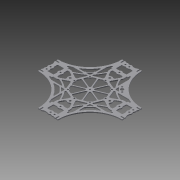
# Autodesk Inventor part: Middle Plate Over
Saved by Autodesk Inventor 2014 SP1 (Build 180222100, 222)
## iProperties
Created: 2014-07-28
Part Number: Middle Plate Over
Material: Generic
Document SubType Name: Modeling
Designer: Ryan
Density: 1 g/cm^3
Appearance: Default
Mass: 14.8472 g
Surface Area: 207.77 cm^2
Volume: 14.8472 cm^3
Author: Ryan
Autodesk Inventor part; units mm, degrees
(part 1 of 2)
ref_plane "YZ Plane" through (0, 0, 0) normal (1, 0, 0) x (0, 1, 0)
ref_plane "XZ Plane" through (0, 0, 0) normal (0, 1, 0) x (-1, 0, 0)
ref_plane "XY Plane" through (0, 0, 0) normal (0, 0, 1) x (1, 0, 0)
sketch "Middle Plate Over" plane through (0, 0, 0) normal (0, 0, 1) x (1, 0, 0)
  circle A0 centre (54.1802, 86) radius 1.6
  circle A1 centre (63.5, 108.5) radius 1.6
  circle A2 centre (86, 117.8198) radius 1.6
  circle A3 centre (108.5, 108.5) radius 1.6
  circle A4 centre (117.8198, 86) radius 1.6
  circle A5 centre (108.5, 63.5) radius 1.6
  circle A6 centre (63.5, 63.5) radius 1.6
  circle A7 centre (86, 54.1802) radius 1.6
  arc A8 (56.1767, 84.1823) -> (56.1767, 87.8177) centre (54.1802, 86) ccw
  arc A9 (55.8078, 89.9295) -> (56.1767, 87.8177) centre (57.6556, 89.1641) ccw
  arc A10 (56.1767, 84.1823) -> (55.8078, 82.0705) centre (57.6556, 82.8359) ccw
  arc A11 (63.6264, 105.803) -> (66.197, 108.3735) centre (63.5, 108.5) ccw
  arc A12 (63.6264, 105.803) -> (61.8724, 104.5705) centre (63.7201, 103.8052) ccw
  arc A13 (67.4295, 110.1276) -> (66.197, 108.3735) centre (68.1948, 108.2799) ccw
  arc A14 (84.1823, 115.8233) -> (87.8177, 115.8233) centre (86, 117.8198) ccw
  arc A15 (89.9295, 116.1922) -> (87.8177, 115.8233) centre (89.1641, 114.3444) ccw
  arc A16 (84.1823, 115.8233) -> (82.0705, 116.1922) centre (82.8359, 114.3444) ccw
  arc A17 (105.803, 108.3735) -> (108.3735, 105.803) centre (108.5, 108.5) ccw
  arc A18 (110.1276, 104.5705) -> (108.3735, 105.803) centre (108.2799, 103.8052) ccw
  arc A19 (105.803, 108.3735) -> (104.5705, 110.1276) centre (103.8052, 108.2799) ccw
  arc A20 (115.8233, 87.8177) -> (115.8233, 84.1823) centre (117.8198, 86) ccw
  arc A21 (116.1922, 82.0705) -> (115.8233, 84.1823) centre (114.3444, 82.8359) ccw
  arc A22 (115.8233, 87.8177) -> (116.1922, 89.9295) centre (114.3444, 89.1641) ccw
  arc A23 (66.197, 63.6265) -> (63.6264, 66.197) centre (63.5, 63.5) ccw
  arc A24 (61.8724, 67.4295) -> (63.6264, 66.197) centre (63.7201, 68.1948) ccw
  arc A25 (66.197, 63.6265) -> (67.4295, 61.8724) centre (68.1948, 63.7201) ccw
  arc A26 (87.8177, 56.1767) -> (84.1823, 56.1767) centre (86, 54.1802) ccw
  arc A27 (82.0705, 55.8078) -> (84.1823, 56.1767) centre (82.8359, 57.6556) ccw
  arc A28 (87.8177, 56.1767) -> (89.9295, 55.8078) centre (89.1641, 57.6556) ccw
  arc A29 (108.3735, 66.197) -> (105.803, 63.6265) centre (108.5, 63.5) ccw
  arc A30 (104.5705, 61.8724) -> (105.803, 63.6265) centre (103.8052, 63.7201) ccw
  arc A31 (108.3735, 66.197) -> (110.1276, 67.4295) centre (108.2799, 68.1948) ccw
  line L0 (55.8078, 82.0705) -> (61.8724, 67.4295)
  line L1 (67.4295, 61.8724) -> (82.0705, 55.8078)
  line L2 (89.9295, 55.8078) -> (104.5705, 61.8724)
  line L3 (110.1276, 67.4295) -> (116.1922, 82.0705)
  line L4 (116.1922, 89.9295) -> (110.1276, 104.5705)
  line L5 (104.5705, 110.1276) -> (89.9295, 116.1922)
  line L6 (82.0705, 116.1922) -> (67.4295, 110.1276)
  line L7 (61.8724, 104.5705) -> (55.8078, 89.9295)
  line L8 (0, 99.484) -> (0, 101)
  arc A32 (0, 99.484) -> (0.217, 98.5779) centre (2, 99.484) ccw
  line L9 (0, 101) -> (6.5, 101)
  line L10 (6.5, 101) -> (6.5, 103.2)
  line L11 (6.5, 103.2) -> (0, 103.2)
  line L12 (0, 103.2) -> (0, 106.2)
  line L13 (71, 172) -> (71, 165.5)
  line L14 (71, 165.5) -> (68.8, 165.5)
  line L15 (68.8, 165.5) -> (68.8, 172)
  line L16 (68.8, 172) -> (65.8, 172)
  arc A33 (0, 106.2) -> (65.8, 172) centre (0, 172) ccw
  line L17 (101, 172) -> (101, 165.5)
  line L18 (101, 165.5) -> (103.2, 165.5)
  line L19 (103.2, 165.5) -> (103.2, 172)
  line L20 (103.2, 172) -> (106.2, 172)
  line L21 (172, 101) -> (165.5, 101)
  line L22 (165.5, 101) -> (165.5, 103.2)
  line L23 (165.5, 103.2) -> (172, 103.2)
  line L24 (172, 103.2) -> (172, 106.2)
  arc A34 (106.2, 172) -> (172, 106.2) centre (172, 172) ccw
  line L25 (0, 71) -> (6.5, 71)
  line L26 (6.5, 71) -> (6.5, 68.8)
  line L27 (6.5, 68.8) -> (0, 68.8)
  line L28 (0, 68.8) -> (0, 65.8)
  line L29 (71, 0) -> (71, 6.5)
  line L30 (71, 6.5) -> (68.8, 6.5)
  line L31 (68.8, 6.5) -> (68.8, 0)
  line L32 (68.8, 0) -> (65.8, 0)
  arc A35 (65.8, 0) -> (0, 65.8) centre (0, 0) ccw
  line L33 (101, 0) -> (101, 6.5)
  line L34 (101, 6.5) -> (103.2, 6.5)
  line L35 (103.2, 6.5) -> (103.2, 0)
  line L36 (103.2, 0) -> (106.2, 0)
  line L37 (172, 71) -> (165.5, 71)
  line L38 (165.5, 71) -> (165.5, 68.8)
  line L39 (165.5, 68.8) -> (172, 68.8)
  line L40 (172, 68.8) -> (172, 65.8)
  arc A36 (172, 65.8) -> (106.2, 0) centre (172, 0) ccw
  circle A37 centre (45.5084, 86) radius 2.1
  circle A38 centre (5.472, 86) radius 1.6
  circle A39 centre (25.7484, 86) radius 1.6
  line L41 (10.792, 96.8671) -> (20.4284, 96.8671)
  arc A40 (10.792, 96.8671) -> (8.892, 94.9671) centre (10.792, 94.9671) ccw
  line L42 (8.892, 94.9671) -> (8.892, 89.42)
  line L43 (22.3284, 89.42) -> (22.3284, 94.9671)
  arc A41 (22.3284, 94.9671) -> (20.4284, 96.8671) centre (20.4284, 94.9671) ccw
  line L44 (10.2433, 75.1329) -> (20.4284, 75.1329)
  line L45 (22.3284, 82.58) -> (22.3284, 77.0329)
  arc A42 (20.4284, 75.1329) -> (22.3284, 77.0329) centre (20.4284, 77.0329) ccw
  arc A43 (9.3838, 83.1636) -> (8.892, 89.42) centre (5.426, 86) ccw
  arc A44 (22.3284, 89.42) -> (22.3284, 82.58) centre (25.7484, 86) ccw
  line L46 (32.9349, 96.8671) -> (31.0684, 96.8671)
  line L47 (29.1684, 89.42) -> (29.1684, 94.9671)
  arc A45 (31.0684, 96.8671) -> (29.1684, 94.9671) centre (31.0684, 94.9671) ccw
  arc A46 (29.1684, 82.58) -> (29.1684, 89.42) centre (25.7484, 86) ccw
  line L48 (33.8405, 96.6374) -> (41.094, 92.7047)
  arc A47 (33.8405, 96.6374) -> (32.9349, 96.8671) centre (32.9349, 94.9671) ccw
  line L49 (42.0884, 91.0344) -> (42.0884, 89.42)
  arc A48 (42.0884, 91.0344) -> (41.094, 92.7047) centre (40.1884, 91.0344) ccw
  arc A49 (42.0884, 89.42) -> (42.0884, 82.58) centre (45.5084, 86) ccw
  line L50 (32.9349, 75.1329) -> (31.0684, 75.1329)
  line L51 (29.1684, 82.58) -> (29.1684, 77.0329)
  arc A50 (29.1684, 77.0329) -> (31.0684, 75.1329) centre (31.0684, 77.0329) ccw
  line L52 (33.8405, 75.3626) -> (41.094, 79.2953)
  arc A51 (32.9349, 75.1329) -> (33.8405, 75.3626) centre (32.9349, 77.0329) ccw
  line L53 (42.0884, 80.9656) -> (42.0884, 82.58)
  arc A52 (41.094, 79.2953) -> (42.0884, 80.9656) centre (40.1884, 80.9656) ccw
  circle A53 centre (126.4916, 86) radius 2.1
  circle A54 centre (146.2516, 86) radius 1.6
  line L54 (161.7567, 96.8671) -> (151.5716, 96.8671)
  line L55 (149.6716, 89.42) -> (149.6716, 94.9671)
  arc A55 (151.5716, 96.8671) -> (149.6716, 94.9671) centre (151.5716, 94.9671) ccw
  line L56 (161.208, 75.1329) -> (151.5716, 75.1329)
  line L57 (149.6716, 82.58) -> (149.6716, 77.0329)
  arc A56 (149.6716, 77.0329) -> (151.5716, 75.1329) centre (151.5716, 77.0329) ccw
  arc A57 (149.6716, 82.58) -> (149.6716, 89.42) centre (146.2516, 86) ccw
  line L58 (139.0651, 96.8671) -> (140.9316, 96.8671)
  line L59 (142.8316, 89.42) -> (142.8316, 94.9671)
  arc A58 (142.8316, 94.9671) -> (140.9316, 96.8671) centre (140.9316, 94.9671) ccw
  arc A59 (142.8316, 89.42) -> (142.8316, 82.58) centre (146.2516, 86) ccw
  line L60 (138.1595, 96.6374) -> (130.906, 92.7047)
  arc A60 (139.0651, 96.8671) -> (138.1595, 96.6374) centre (139.0651, 94.9671) ccw
  line L61 (129.9116, 91.0344) -> (129.9116, 89.42)
  arc A61 (130.906, 92.7047) -> (129.9116, 91.0344) centre (131.8116, 91.0344) ccw
  arc A62 (129.9116, 82.58) -> (129.9116, 89.42) centre (126.4916, 86) ccw
  line L62 (139.0651, 75.1329) -> (140.9316, 75.1329)
  line L63 (142.8316, 82.58) -> (142.8316, 77.0329)
  arc A63 (140.9316, 75.1329) -> (142.8316, 77.0329) centre (140.9316, 77.0329) ccw
  line L64 (138.1595, 75.3626) -> (130.906, 79.2953)
  arc A64 (138.1595, 75.3626) -> (139.0651, 75.1329) centre (139.0651, 77.0329) ccw
  line L65 (129.9116, 80.9656) -> (129.9116, 82.58)
  arc A65 (129.9116, 80.9656) -> (130.906, 79.2953) centre (131.8116, 80.9656) ccw
  circle A66 centre (86, 126.4916) radius 2.1
  circle A67 centre (86, 146.2516) radius 1.6
  line L66 (75.1329, 161.7567) -> (75.1329, 151.5716)
  line L67 (82.58, 149.6716) -> (77.0329, 149.6716)
  arc A68 (75.1329, 151.5716) -> (77.0329, 149.6716) centre (77.0329, 151.5716) ccw
  line L68 (96.8671, 161.208) -> (96.8671, 151.5716)
  line L69 (89.42, 149.6716) -> (94.9671, 149.6716)
  arc A69 (94.9671, 149.6716) -> (96.8671, 151.5716) centre (94.9671, 151.5716) ccw
  arc A70 (89.42, 149.6716) -> (82.58, 149.6716) centre (86, 146.2516) ccw
  line L70 (75.1329, 139.0651) -> (75.1329, 140.9316)
  line L71 (82.58, 142.8316) -> (77.0329, 142.8316)
  arc A71 (77.0329, 142.8316) -> (75.1329, 140.9316) centre (77.0329, 140.9316) ccw
  arc A72 (82.58, 142.8316) -> (89.42, 142.8316) centre (86, 146.2516) ccw
  line L72 (75.3626, 138.1595) -> (79.2953, 130.906)
  arc A73 (75.1329, 139.0651) -> (75.3626, 138.1595) centre (77.0329, 139.0651) ccw
  arc A74 (96.8671, 20.4284) -> (94.9671, 22.3284) centre (94.9671, 20.4284) ccw
  line L73 (80.9656, 129.9116) -> (82.58, 129.9116)
  arc A75 (79.2953, 130.906) -> (80.9656, 129.9116) centre (80.9656, 131.8116) ccw
  arc A76 (89.42, 129.9116) -> (82.58, 129.9116) centre (86, 126.4916) ccw
  line L74 (96.8671, 139.0651) -> (96.8671, 140.9316)
  line L75 (89.42, 142.8316) -> (94.9671, 142.8316)
  arc A77 (96.8671, 140.9316) -> (94.9671, 142.8316) centre (94.9671, 140.9316) ccw
  line L76 (96.6374, 138.1595) -> (92.7047, 130.906)
  line L77 (96.8671, 32.9349) -> (96.8671, 31.0684)
  arc A78 (96.6374, 138.1595) -> (96.8671, 139.0651) centre (94.9671, 139.0651) ccw
  line L78 (91.0344, 129.9116) -> (89.42, 129.9116)
  arc A79 (91.0344, 129.9116) -> (92.7047, 130.906) centre (91.0344, 131.8116) ccw
  circle A80 centre (86, 45.5084) radius 2.1
  circle A81 centre (86, 25.7484) radius 1.6
  line L79 (96.8671, 10.2433) -> (96.8671, 20.4284)
  line L80 (89.42, 22.3284) -> (94.9671, 22.3284)
  line L81 (75.1329, 10.792) -> (75.1329, 20.4284)
  arc A82 (92.7047, 41.094) -> (91.0344, 42.0884) centre (91.0344, 40.1884) ccw
  line L82 (82.58, 22.3284) -> (77.0329, 22.3284)
  line L83 (82.58, 29.1684) -> (77.0329, 29.1684)
  arc A83 (77.0329, 22.3284) -> (75.1329, 20.4284) centre (77.0329, 20.4284) ccw
  arc A84 (82.58, 22.3284) -> (89.42, 22.3284) centre (86, 25.7484) ccw
  line L84 (80.9656, 42.0884) -> (82.58, 42.0884)
  line L85 (89.42, 29.1684) -> (94.9671, 29.1684)
  arc A85 (94.9671, 29.1684) -> (96.8671, 31.0684) centre (94.9671, 31.0684) ccw
  arc A86 (89.42, 29.1684) -> (82.58, 29.1684) centre (86, 25.7484) ccw
  line L86 (96.6374, 33.8405) -> (92.7047, 41.094)
  arc A87 (96.8671, 32.9349) -> (96.6374, 33.8405) centre (94.9671, 32.9349) ccw
  line L87 (91.0344, 42.0884) -> (89.42, 42.0884)
  arc A88 (82.58, 42.0884) -> (89.42, 42.0884) centre (86, 45.5084) ccw
  line L88 (75.1329, 32.9349) -> (75.1329, 31.0684)
  arc A89 (75.1329, 31.0684) -> (77.0329, 29.1684) centre (77.0329, 31.0684) ccw
  arc A90 (80.9656, 42.0884) -> (79.2953, 41.094) centre (80.9656, 40.1884) ccw
  line L89 (75.3626, 33.8405) -> (79.2953, 41.094)
  arc A91 (75.3626, 33.8405) -> (75.1329, 32.9349) centre (77.0329, 32.9349) ccw
  line L90 (2.052, 94.4881) -> (2.052, 89.42)
  arc A92 (2.052, 89.42) -> (1.5587, 83.1656) centre (5.518, 86) ccw
  line L91 (0.217, 98.5779) -> (1.835, 95.3941)
  arc A93 (2.052, 94.4881) -> (1.835, 95.3941) centre (0.052, 94.4881) ccw
  arc A94 (0.217, 73.4221) -> (0, 72.516) centre (2, 72.516) ccw
  line L92 (0.217, 73.4221) -> (0.8629, 74.6931)
  line L93 (0, 71) -> (0, 72.516)
  circle A95 centre (5.47, 78) radius 1.6
  arc A96 (9.7945, 75.8533) -> (9.3832, 80.8344) centre (5.424, 78) ccw
  arc A97 (9.7945, 75.8533) -> (10.2433, 75.1329) centre (10.2433, 75.6329) ccw
  arc A98 (9.3838, 83.1636) -> (9.3832, 80.8344) centre (11.0095, 81.9986) ccw
  arc A99 (1.5581, 80.8364) -> (0.9538, 76.2982) centre (5.516, 78) ccw
  arc A100 (1.5581, 80.8364) -> (1.5587, 83.1656) centre (-0.0675, 82.0014) ccw
  arc A101 (0.8629, 74.6931) -> (0.9538, 76.2982) centre (-0.9201, 75.5992) ccw
  line L94 (172, 72.516) -> (172, 71)
  arc A102 (172, 72.516) -> (171.783, 73.4221) centre (170, 72.516) ccw
  circle A103 centre (166.528, 86) radius 1.6
  arc A104 (161.208, 75.1329) -> (163.108, 77.0329) centre (161.208, 77.0329) ccw
  line L95 (163.108, 77.0329) -> (163.108, 82.58)
  arc A105 (162.6162, 88.8364) -> (163.108, 82.58) centre (166.574, 86) ccw
  line L96 (169.948, 77.5119) -> (169.948, 82.58)
  arc A106 (169.948, 82.58) -> (170.4413, 88.8344) centre (166.482, 86) ccw
  line L97 (171.783, 73.4221) -> (170.165, 76.6059)
  arc A107 (169.948, 77.5119) -> (170.165, 76.6059) centre (171.948, 77.5119) ccw
  arc A108 (171.783, 98.5779) -> (172, 99.484) centre (170, 99.484) ccw
  line L98 (171.783, 98.5779) -> (171.1371, 97.3069)
  line L99 (172, 101) -> (172, 99.484)
  circle A109 centre (166.53, 94) radius 1.6
  arc A110 (162.2055, 96.1467) -> (162.6167, 91.1656) centre (166.576, 94) ccw
  arc A111 (162.2055, 96.1467) -> (161.7567, 96.8671) centre (161.7567, 96.3671) ccw
  arc A112 (162.6162, 88.8364) -> (162.6167, 91.1656) centre (160.9905, 90.0014) ccw
  arc A113 (170.4419, 91.1636) -> (171.0462, 95.7018) centre (166.484, 94) ccw
  arc A114 (170.4419, 91.1636) -> (170.4413, 88.8344) centre (172.0675, 89.9986) ccw
  arc A115 (171.1371, 97.3069) -> (171.0462, 95.7018) centre (172.92, 96.4008) ccw
  line L100 (72.516, 0) -> (71, 0)
  arc A116 (72.516, 0) -> (73.4221, 0.217) centre (72.516, 2) ccw
  circle A117 centre (86, 5.472) radius 1.6
  arc A118 (75.1329, 10.792) -> (77.0329, 8.892) centre (77.0329, 10.792) ccw
  line L101 (77.0329, 8.892) -> (82.58, 8.892)
  arc A119 (88.8364, 9.3838) -> (82.58, 8.892) centre (86, 5.426) ccw
  line L102 (77.5119, 2.052) -> (82.58, 2.052)
  arc A120 (82.58, 2.052) -> (88.8344, 1.5587) centre (86, 5.518) ccw
  line L103 (73.4221, 0.217) -> (76.6059, 1.835)
  arc A121 (77.5119, 2.052) -> (76.6059, 1.835) centre (77.5119, 0.052) ccw
  arc A122 (98.5779, 0.217) -> (99.484, 0) centre (99.484, 2) ccw
  line L104 (98.5779, 0.217) -> (97.3069, 0.8629)
  line L105 (101, 0) -> (99.484, 0)
  circle A123 centre (94, 5.47) radius 1.6
  arc A124 (96.1467, 9.7945) -> (91.1656, 9.3833) centre (94, 5.424) ccw
  arc A125 (96.1467, 9.7945) -> (96.8671, 10.2433) centre (96.3671, 10.2433) ccw
  arc A126 (88.8364, 9.3838) -> (91.1656, 9.3833) centre (90.0014, 11.0095) ccw
  arc A127 (91.1636, 1.5581) -> (95.7018, 0.9538) centre (94, 5.516) ccw
  arc A128 (91.1636, 1.5581) -> (88.8344, 1.5587) centre (89.9986, -0.0675) ccw
  arc A129 (97.3069, 0.8629) -> (95.7018, 0.9538) centre (96.4008, -0.92) ccw
  line L106 (99.484, 172) -> (101, 172)
  arc A130 (99.484, 172) -> (98.5779, 171.783) centre (99.484, 170) ccw
  circle A131 centre (86, 166.528) radius 1.6
  arc A132 (96.8671, 161.208) -> (94.9671, 163.108) centre (94.9671, 161.208) ccw
  line L107 (94.9671, 163.108) -> (89.42, 163.108)
  arc A133 (83.1636, 162.6162) -> (89.42, 163.108) centre (86, 166.574) ccw
  line L108 (94.4881, 169.948) -> (89.42, 169.948)
  arc A134 (89.42, 169.948) -> (83.1656, 170.4413) centre (86, 166.482) ccw
  line L109 (98.5779, 171.783) -> (95.3941, 170.165)
  arc A135 (94.4881, 169.948) -> (95.3941, 170.165) centre (94.4881, 171.948) ccw
  arc A136 (73.4221, 171.783) -> (72.516, 172) centre (72.516, 170) ccw
  line L110 (73.4221, 171.783) -> (74.6931, 171.1371)
  line L111 (71, 172) -> (72.516, 172)
  circle A137 centre (78, 166.53) radius 1.6
  arc A138 (75.8533, 162.2055) -> (80.8344, 162.6167) centre (78, 166.576) ccw
  arc A139 (75.8533, 162.2055) -> (75.1329, 161.7567) centre (75.6329, 161.7567) ccw
  arc A140 (83.1636, 162.6162) -> (80.8344, 162.6167) centre (81.9986, 160.9905) ccw
  arc A141 (80.8364, 170.4419) -> (76.2982, 171.0462) centre (78, 166.484) ccw
  arc A142 (80.8364, 170.4419) -> (83.1656, 170.4413) centre (82.0014, 172.0675) ccw
  arc A143 (74.6931, 171.1371) -> (76.2982, 171.0462) centre (75.5992, 172.92) ccw
  arc A144 (38.545, 113.3432) -> (58.6568, 133.455) centre (3.1615, 168.8384) ccw
  arc A145 (38.545, 113.3432) -> (39.0827, 111.5) centre (39.0827, 112.5) ccw
  arc A146 (60.5, 132.9173) -> (58.6568, 133.455) centre (59.5, 132.9173) ccw
  line L112 (58, 111.5) -> (53.3233, 111.5)
  line L113 (48.0955, 111.5) -> (39.0827, 111.5)
  line L114 (60.5, 114) -> (60.5, 118.6767)
  line L115 (60.5, 123.9045) -> (60.5, 132.9173)
  arc A147 (58, 111.5) -> (60.5, 114) centre (58, 114) ccw
  circle A148 centre (53.1485, 53.0665) radius 3.15
  circle A149 centre (48.4963, 57.6887) radius 1.6
  circle A150 centre (57.6887, 48.4963) radius 1.6
  line L116 (63.5, 122.7047) -> (63.5, 142.036)
  arc A151 (63.7361, 116.072) -> (73.3555, 131.2701) centre (13.4685, 158.5315) ccw
  arc A152 (63.7361, 116.072) -> (63.5, 115.4267) centre (64.5, 115.4267) ccw
  arc A153 (75.1447, 131.3324) -> (73.3555, 131.2701) centre (74.2656, 130.8558) ccw
  arc A154 (63.7004, 143.0168) -> (65.9031, 148.9586) centre (3.1615, 168.8384) ccw
  arc A155 (63.7004, 143.0168) -> (63.5, 142.036) centre (66, 142.036) ccw
  arc A156 (68.8, 150.6725) -> (65.9031, 148.9586) centre (68.4135, 148.0207) ccw
  line L117 (71.3627, 138.308) -> (72.3159, 136.55)
  line L118 (71, 146.5) -> (71, 139.7379)
  arc A157 (71, 139.7379) -> (71.3627, 138.308) centre (74, 139.7379) ccw
  arc A158 (49.3372, 111.9321) -> (60.0679, 122.6628) centre (8.4853, 163.5147) ccw
  arc A159 (48.0955, 111.5) -> (49.3372, 111.9321) centre (48.0955, 113.5) ccw
  arc A160 (60.0679, 122.6628) -> (60.5, 123.9045) centre (58.5, 123.9045) ccw
  arc A161 (52.9958, 112.3778) -> (59.6222, 119.0042) centre (9.8995, 162.1005) ccw
  arc A162 (52.9958, 112.3778) -> (53.3233, 111.5) centre (53.3233, 112) ccw
  arc A163 (60.5, 118.6767) -> (59.6222, 119.0042) centre (60, 118.6767) ccw
  arc A164 (113.3432, 133.455) -> (133.455, 113.3432) centre (168.8384, 168.8384) ccw
  arc A165 (132.9173, 111.5) -> (133.455, 113.3432) centre (132.9173, 112.5) ccw
  arc A166 (113.3432, 133.455) -> (111.5, 132.9173) centre (112.5, 132.9173) ccw
  line L119 (114, 111.5) -> (118.6767, 111.5)
  line L120 (123.9045, 111.5) -> (132.9173, 111.5)
  line L121 (111.5, 114) -> (111.5, 118.6767)
  line L122 (111.5, 123.9045) -> (111.5, 132.9173)
  arc A167 (111.5, 114) -> (114, 111.5) centre (114, 114) ccw
  arc A168 (111.9321, 122.6628) -> (122.6628, 111.9321) centre (163.5147, 163.5147) ccw
  arc A169 (122.6628, 111.9321) -> (123.9045, 111.5) centre (123.9045, 113.5) ccw
  arc A170 (111.5, 123.9045) -> (111.9321, 122.6628) centre (113.5, 123.9045) ccw
  arc A171 (112.3778, 119.0042) -> (119.0041, 112.3778) centre (162.1005, 162.1005) ccw
  arc A172 (118.6767, 111.5) -> (119.0041, 112.3778) centre (118.6767, 112) ccw
  arc A173 (112.3778, 119.0042) -> (111.5, 118.6767) centre (112, 118.6767) ccw
  arc A174 (133.455, 58.6568) -> (113.3432, 38.545) centre (168.8384, 3.1616) ccw
  arc A175 (133.455, 58.6568) -> (132.9173, 60.5) centre (132.9173, 59.5) ccw
  arc A176 (111.5, 39.0827) -> (113.3432, 38.545) centre (112.5, 39.0827) ccw
  line L123 (114, 60.5) -> (118.6767, 60.5)
  line L124 (123.9045, 60.5) -> (132.9173, 60.5)
  line L125 (111.5, 58) -> (111.5, 53.3233)
  line L126 (111.5, 48.0955) -> (111.5, 39.0827)
  arc A177 (114, 60.5) -> (111.5, 58) centre (114, 58) ccw
  arc A178 (122.6628, 60.0679) -> (111.9321, 49.3372) centre (163.5147, 8.4853) ccw
  arc A179 (123.9045, 60.5) -> (122.6628, 60.0679) centre (123.9045, 58.5) ccw
  arc A180 (111.9321, 49.3372) -> (111.5, 48.0955) centre (113.5, 48.0955) ccw
  arc A181 (119.0041, 59.6222) -> (112.3778, 52.9958) centre (162.1005, 9.8995) ccw
  arc A182 (119.0041, 59.6222) -> (118.6767, 60.5) centre (118.6767, 60) ccw
  arc A183 (111.5, 53.3233) -> (112.3778, 52.9958) centre (112, 53.3233) ccw
  line L127 (58, 60.5) -> (53.3233, 60.5)
  line L128 (60.5, 58) -> (60.5, 53.3233)
  arc A184 (60.5, 58) -> (58, 60.5) centre (58, 58) ccw
  arc A185 (59.6222, 52.9958) -> (52.9958, 59.6222) centre (9.8995, 9.8995) ccw
  arc A186 (53.3233, 60.5) -> (52.9958, 59.6222) centre (53.3233, 60) ccw
  arc A187 (59.6222, 52.9958) -> (60.5, 53.3233) centre (60, 53.3233) ccw
  line L129 (75.1447, 131.3324) -> (80.089, 122.2131)
  arc A188 (78.848, 118.7118) -> (80.089, 122.2131) centre (77.8913, 121.0215) ccw
  line L130 (64.8827, 112.9272) -> (78.848, 118.7118)
  arc A189 (65.314, 122.1239) -> (72.401, 134.8209) centre (11.7536, 160.3459) ccw
  arc A190 (63.5, 122.7047) -> (65.314, 122.1239) centre (64.5, 122.7047) ccw
  arc A191 (72.401, 134.8209) -> (72.3159, 136.55) centre (70.5576, 135.5967) ccw
  line L131 (63.5, 115.4267) -> (63.5, 113.8511)
  arc A192 (63.5, 113.8511) -> (64.8827, 112.9272) centre (64.5, 113.8511) ccw
  line L132 (49.2953, 108.5) -> (29.964, 108.5)
  arc A193 (40.7299, 98.6445) -> (55.928, 108.2639) centre (13.4685, 158.5315) ccw
  arc A194 (56.5733, 108.5) -> (55.928, 108.2639) centre (56.5733, 107.5) ccw
  arc A195 (40.7299, 98.6445) -> (40.6676, 96.8553) centre (41.1442, 97.7344) ccw
  arc A196 (23.0414, 106.0969) -> (28.9832, 108.2996) centre (3.1615, 168.8384) ccw
  arc A197 (29.964, 108.5) -> (28.9832, 108.2996) centre (29.964, 106) ccw
  arc A198 (23.0414, 106.0969) -> (21.3275, 103.2) centre (23.9793, 103.5865) ccw
  line L133 (33.692, 100.6373) -> (35.45, 99.6841)
  line L134 (25.5, 101) -> (32.2621, 101)
  arc A199 (33.692, 100.6373) -> (32.2621, 101) centre (32.2621, 98) ccw
  line L135 (40.6676, 96.8553) -> (49.7869, 91.911)
  arc A200 (49.7869, 91.911) -> (53.2882, 93.152) centre (50.9785, 94.1087) ccw
  line L136 (59.0728, 107.1173) -> (53.2882, 93.152)
  arc A201 (37.1791, 99.599) -> (49.8761, 106.686) centre (11.6541, 160.2464) ccw
  arc A202 (49.8761, 106.686) -> (49.2953, 108.5) centre (49.2953, 107.5) ccw
  arc A203 (35.45, 99.6841) -> (37.1791, 99.599) centre (36.4033, 101.4424) ccw
  line L137 (56.5733, 108.5) -> (58.1489, 108.5)
  arc A204 (59.0728, 107.1173) -> (58.1489, 108.5) centre (58.1489, 107.5) ccw
  line L138 (122.7047, 63.5) -> (142.036, 63.5)
  arc A205 (131.2701, 73.3555) -> (116.072, 63.7361) centre (158.5315, 13.4685) ccw
  arc A206 (115.4267, 63.5) -> (116.072, 63.7361) centre (115.4267, 64.5) ccw
  arc A207 (131.2701, 73.3555) -> (131.3324, 75.1447) centre (130.8558, 74.2656) ccw
  arc A208 (148.9586, 65.9031) -> (143.0168, 63.7004) centre (168.8384, 3.1616) ccw
  arc A209 (142.036, 63.5) -> (143.0168, 63.7004) centre (142.036, 66) ccw
  arc A210 (148.9586, 65.9031) -> (150.6725, 68.8) centre (148.0207, 68.4135) ccw
  line L139 (138.308, 71.3627) -> (136.55, 72.3159)
  line L140 (146.5, 71) -> (139.7379, 71)
  arc A211 (138.308, 71.3627) -> (139.7379, 71) centre (139.7379, 74) ccw
  line L141 (131.3324, 75.1447) -> (122.2131, 80.089)
  arc A212 (122.2131, 80.089) -> (118.7118, 78.848) centre (121.0215, 77.8913) ccw
  line L142 (112.9272, 64.8827) -> (118.7118, 78.848)
  arc A213 (134.8209, 72.401) -> (122.1239, 65.314) centre (160.3459, 11.7536) ccw
  arc A214 (122.1239, 65.314) -> (122.7047, 63.5) centre (122.7047, 64.5) ccw
  arc A215 (136.55, 72.3159) -> (134.8209, 72.401) centre (135.5967, 70.5576) ccw
  line L143 (115.4267, 63.5) -> (113.8511, 63.5)
  arc A216 (112.9272, 64.8827) -> (113.8511, 63.5) centre (113.8511, 64.5) ccw
  line L144 (108.5, 49.2953) -> (108.5, 29.964)
  arc A217 (108.2639, 55.928) -> (98.6445, 40.7299) centre (158.5315, 13.4685) ccw
  arc A218 (108.2639, 55.928) -> (108.5, 56.5733) centre (107.5, 56.5733) ccw
  arc A219 (96.8553, 40.6676) -> (98.6445, 40.7299) centre (97.7344, 41.1442) ccw
  arc A220 (108.2996, 28.9832) -> (106.0968, 23.0414) centre (168.8384, 3.1616) ccw
  arc A221 (108.2996, 28.9832) -> (108.5, 29.964) centre (106, 29.964) ccw
  arc A222 (103.2, 21.3275) -> (106.0968, 23.0414) centre (103.5865, 23.9793) ccw
  line L145 (100.6373, 33.692) -> (99.6841, 35.45)
  line L146 (101, 25.5) -> (101, 32.2621)
  arc A223 (101, 32.2621) -> (100.6373, 33.692) centre (98, 32.2621) ccw
  line L147 (96.8553, 40.6676) -> (91.911, 49.7869)
  arc A224 (93.152, 53.2882) -> (91.911, 49.7869) centre (94.1087, 50.9785) ccw
  line L148 (107.1173, 59.0728) -> (93.152, 53.2882)
  arc A225 (106.686, 49.8761) -> (99.599, 37.1791) centre (160.2464, 11.6541) ccw
  arc A226 (108.5, 49.2953) -> (106.686, 49.8761) centre (107.5, 49.2953) ccw
  arc A227 (99.599, 37.1791) -> (99.6841, 35.45) centre (101.4423, 36.4033) ccw
  line L149 (108.5, 56.5733) -> (108.5, 58.1489)
  arc A228 (108.5, 58.1489) -> (107.1173, 59.0728) centre (107.5, 58.1489) ccw
  line L150 (63.5, 49.2953) -> (63.5, 29.964)
  arc A229 (73.3555, 40.7299) -> (63.7361, 55.928) centre (13.4685, 13.4685) ccw
  arc A230 (63.5, 56.5733) -> (63.7361, 55.928) centre (64.5, 56.5733) ccw
  arc A231 (73.3555, 40.7299) -> (75.1447, 40.6676) centre (74.2656, 41.1442) ccw
  arc A232 (65.9031, 23.0414) -> (63.7004, 28.9832) centre (3.1615, 3.1616) ccw
  arc A233 (63.5, 29.964) -> (63.7004, 28.9832) centre (66, 29.964) ccw
  arc A234 (65.9031, 23.0414) -> (68.8, 21.3275) centre (68.4135, 23.9793) ccw
  line L151 (71.3627, 33.692) -> (72.3159, 35.45)
  line L152 (71, 25.5) -> (71, 32.2621)
  arc A235 (71.3627, 33.692) -> (71, 32.2621) centre (74, 32.2621) ccw
  line L153 (75.1447, 40.6676) -> (80.089, 49.7869)
  arc A236 (80.089, 49.7869) -> (78.848, 53.2882) centre (77.8913, 50.9785) ccw
  line L154 (64.8827, 59.0728) -> (78.848, 53.2882)
  arc A237 (72.401, 37.1791) -> (65.314, 49.8761) centre (11.7536, 11.6541) ccw
  arc A238 (65.314, 49.8761) -> (63.5, 49.2953) centre (64.5, 49.2953) ccw
  arc A239 (72.3159, 35.45) -> (72.401, 37.1791) centre (70.5576, 36.4033) ccw
  line L155 (63.5, 56.5733) -> (63.5, 58.1489)
  arc A240 (64.8827, 59.0728) -> (63.5, 58.1489) centre (64.5, 58.1489) ccw
  line L156 (49.2953, 63.5) -> (29.964, 63.5)
  arc A241 (55.928, 63.7361) -> (40.7299, 73.3555) centre (13.4685, 13.4685) ccw
  arc A242 (55.928, 63.7361) -> (56.5733, 63.5) centre (56.5733, 64.5) ccw
  arc A243 (40.6676, 75.1447) -> (40.7299, 73.3555) centre (41.1442, 74.2656) ccw
  arc A244 (28.9832, 63.7004) -> (23.0414, 65.9031) centre (3.1615, 3.1616) ccw
  arc A245 (28.9832, 63.7004) -> (29.964, 63.5) centre (29.964, 66) ccw
  arc A246 (21.3275, 68.8) -> (23.0414, 65.9031) centre (23.9793, 68.4135) ccw
  line L157 (33.692, 71.3627) -> (35.45, 72.3159)
  line L158 (25.5, 71) -> (32.2621, 71)
  arc A247 (32.2621, 71) -> (33.692, 71.3627) centre (32.2621, 74) ccw
  line L159 (40.6676, 75.1447) -> (49.7869, 80.089)
  arc A248 (53.2882, 78.848) -> (49.7869, 80.089) centre (50.9785, 77.8913) ccw
  line L160 (59.0728, 64.8827) -> (53.2882, 78.848)
  arc A249 (49.8761, 65.314) -> (37.1791, 72.401) centre (11.6541, 11.7536) ccw
  arc A250 (49.2953, 63.5) -> (49.8761, 65.314) centre (49.2953, 64.5) ccw
  arc A251 (37.1791, 72.401) -> (35.45, 72.3159) centre (36.4033, 70.5576) ccw
  line L161 (56.5733, 63.5) -> (58.1489, 63.5)
  arc A252 (58.1489, 63.5) -> (59.0728, 64.8827) centre (58.1489, 64.5) ccw
  line L162 (108.5, 122.7047) -> (108.5, 142.036)
  arc A253 (98.6445, 131.2701) -> (108.2639, 116.072) centre (158.5315, 158.5315) ccw
  arc A254 (108.5, 115.4267) -> (108.2639, 116.072) centre (107.5, 115.4267) ccw
  arc A255 (98.6445, 131.2701) -> (96.8553, 131.3324) centre (97.7344, 130.8558) ccw
  arc A256 (106.0968, 148.9586) -> (108.2996, 143.0168) centre (168.8384, 168.8384) ccw
  arc A257 (108.5, 142.036) -> (108.2996, 143.0168) centre (106, 142.036) ccw
  arc A258 (106.0968, 148.9586) -> (103.2, 150.6725) centre (103.5865, 148.0207) ccw
  line L163 (100.6373, 138.308) -> (99.6841, 136.55)
  line L164 (101, 146.5) -> (101, 139.7379)
  arc A259 (100.6373, 138.308) -> (101, 139.7379) centre (98, 139.7379) ccw
  line L165 (96.8553, 131.3324) -> (91.911, 122.2131)
  arc A260 (91.911, 122.2131) -> (93.152, 118.7118) centre (94.1087, 121.0215) ccw
  line L166 (107.1173, 112.9272) -> (93.152, 118.7118)
  arc A261 (99.599, 134.8209) -> (106.686, 122.1239) centre (160.2464, 160.3459) ccw
  arc A262 (106.686, 122.1239) -> (108.5, 122.7047) centre (107.5, 122.7047) ccw
  arc A263 (99.6841, 136.55) -> (99.599, 134.8209) centre (101.4423, 135.5967) ccw
  line L167 (108.5, 115.4267) -> (108.5, 113.8511)
  arc A264 (107.1173, 112.9272) -> (108.5, 113.8511) centre (107.5, 113.8511) ccw
  line L168 (122.7047, 108.5) -> (142.036, 108.5)
  arc A265 (116.072, 108.2639) -> (131.2701, 98.6445) centre (158.5315, 158.5315) ccw
  arc A266 (116.072, 108.2639) -> (115.4267, 108.5) centre (115.4267, 107.5) ccw
  arc A267 (131.3324, 96.8553) -> (131.2701, 98.6445) centre (130.8558, 97.7344) ccw
  arc A268 (143.0168, 108.2996) -> (148.9586, 106.0969) centre (168.8384, 168.8384) ccw
  arc A269 (143.0168, 108.2996) -> (142.036, 108.5) centre (142.036, 106) ccw
  arc A270 (150.6725, 103.2) -> (148.9586, 106.0969) centre (148.0207, 103.5865) ccw
  line L169 (138.308, 100.6373) -> (136.55, 99.6841)
  line L170 (146.5, 101) -> (139.7379, 101)
  arc A271 (139.7379, 101) -> (138.308, 100.6373) centre (139.7379, 98) ccw
  line L171 (131.3324, 96.8553) -> (122.2131, 91.911)
  arc A272 (118.7118, 93.152) -> (122.2131, 91.911) centre (121.0215, 94.1087) ccw
  line L172 (112.9272, 107.1173) -> (118.7118, 93.152)
  arc A273 (122.1239, 106.686) -> (134.8209, 99.599) centre (160.3459, 160.2464) ccw
  arc A274 (122.7047, 108.5) -> (122.1239, 106.686) centre (122.7047, 107.5) ccw
  arc A275 (134.8209, 99.599) -> (136.55, 99.6841) centre (135.5967, 101.4424) ccw
  line L173 (115.4267, 108.5) -> (113.8511, 108.5)
  arc A276 (113.8511, 108.5) -> (112.9272, 107.1173) centre (113.8511, 107.5) ccw
  line L174 (21.3275, 103.2) -> (25.5, 103.2)
  line L175 (25.5, 103.2) -> (25.5, 101)
  line L176 (21.3275, 68.8) -> (25.5, 68.8)
  line L177 (25.5, 68.8) -> (25.5, 71)
  line L178 (150.6725, 103.2) -> (146.5, 103.2)
  line L179 (146.5, 103.2) -> (146.5, 101)
  line L180 (150.6725, 68.8) -> (146.5, 68.8)
  line L181 (146.5, 68.8) -> (146.5, 71)
  line L182 (68.8, 150.6725) -> (68.8, 146.5)
  line L183 (68.8, 146.5) -> (71, 146.5)
  line L184 (103.2, 150.6725) -> (103.2, 146.5)
  line L185 (103.2, 146.5) -> (101, 146.5)
  line L186 (68.8, 21.3275) -> (68.8, 25.5)
  line L187 (68.8, 25.5) -> (71, 25.5)
  line L188 (103.2, 21.3275) -> (103.2, 25.5)
  line L189 (103.2, 25.5) -> (101, 25.5)
  point P0 (86.5788, 86.5787)
sketch "Sketch1" plane through (0, 0, 0) normal (0, 1, 0) x (-1, 0, 0)
  circle A0 centre (5.472, 86) radius 1.6
  circle A1 centre (25.7484, 86) radius 1.6
  circle A2 centre (5.47, 78) radius 1.6
  circle A3 centre (53.1485, 53.0665) radius 3.15
  circle A4 centre (57.6887, 48.4963) radius 1.6
  circle A5 centre (48.4963, 57.6887) radius 1.6
  circle A6 centre (45.5084, 86) radius 2.1
  circle A7 centre (54.1802, 86) radius 1.6
  circle A8 centre (63.5, 108.5) radius 1.6
  circle A9 centre (63.5, 63.5) radius 1.6
  circle A10 centre (86, 54.1802) radius 1.6
  circle A11 centre (86, 45.5084) radius 2.1
  circle A12 centre (86, 25.7484) radius 1.6027
  circle A13 centre (86, 5.472) radius 1.6
  circle A14 centre (94, 5.47) radius 1.6
  circle A15 centre (108.5, 63.5) radius 1.6
  circle A16 centre (117.8198, 86) radius 1.6
  circle A17 centre (126.4916, 86) radius 2.1
  circle A18 centre (146.2516, 86) radius 1.6
  circle A19 centre (166.528, 86) radius 1.6
  circle A20 centre (166.53, 94) radius 1.6
  circle A21 centre (108.5, 108.5) radius 1.6
  circle A22 centre (86, 117.8198) radius 1.6
  circle A23 centre (86, 126.4916) radius 2.1
  circle A24 centre (86, 146.2516) radius 1.6
  circle A25 centre (78, 166.53) radius 1.6
  circle A26 centre (86, 166.528) radius 1.6
  line L0 (0, 65.8) -> (0, 68.8)
  line L1 (0, 68.8) -> (6.5, 68.8)
  line L2 (6.5, 68.8) -> (6.5, 71)
  line L3 (6.5, 71) -> (0, 71)
  line L4 (0, 71) -> (0, 72.516)
  line L5 (2.052, 89.42) -> (2.052, 94.4881)
  line L6 (0, 101) -> (0, 99.484)
  line L7 (0, 101) -> (6.5, 101)
  line L8 (6.5, 101) -> (6.5, 103.2)
  line L9 (6.5, 103.2) -> (0, 103.2)
  line L10 (0, 103.2) -> (0, 106.2)
  arc A27 (0.217, 73.4221) -> (0, 72.4832) centre (2.0042, 72.5145) ccw
  line L11 (0.8629, 74.6931) -> (0.217, 73.4221)
  arc A28 (0.8629, 74.6931) -> (1.026, 76.0607) centre (-0.9201, 75.5992) ccw
  arc A29 (1.5581, 80.8364) -> (0.9538, 76.2982) centre (5.516, 78) ccw
  arc A30 (1.026, 76.0607) -> (0.9538, 76.2982) centre (-0.9201, 75.5992) ccw
  arc A31 (1.5581, 80.8364) -> (1.5587, 83.1656) centre (-0.0675, 82.0014) ccw
  arc A32 (2.052, 89.42) -> (1.5587, 83.1656) centre (5.518, 86) ccw
  arc A33 (0, 99.484) -> (0.217, 98.5779) centre (2, 99.484) ccw
  arc A34 (2.052, 94.4881) -> (1.835, 95.3941) centre (0.052, 94.4881) ccw
  line L12 (1.835, 95.3941) -> (0.217, 98.5779)
  arc A35 (9.7945, 75.8533) -> (10.2433, 75.1329) centre (10.2433, 75.6329) ccw
  arc A36 (20.4284, 75.1329) -> (22.3284, 77.0329) centre (20.4284, 77.0329) ccw
  arc A37 (10.792, 96.8671) -> (8.892, 94.9671) centre (10.792, 94.9671) ccw
  arc A38 (22.3284, 94.9671) -> (20.4284, 96.8671) centre (20.4284, 94.9671) ccw
  arc A39 (22.3284, 89.42) -> (22.3284, 82.58) centre (25.7484, 86) ccw
  arc A40 (29.1684, 82.58) -> (29.1684, 89.42) centre (25.7484, 86) ccw
  line L13 (22.3284, 82.58) -> (22.3284, 77.0329)
  line L14 (20.4284, 75.1329) -> (10.2433, 75.1329)
  arc A41 (9.7945, 75.8533) -> (9.3832, 80.8344) centre (5.424, 78) ccw
  arc A42 (9.3838, 83.1636) -> (9.3832, 80.8344) centre (11.0095, 81.9986) ccw
  arc A43 (9.3838, 83.1636) -> (8.892, 89.42) centre (5.426, 86) ccw
  line L15 (10.792, 96.8671) -> (20.4284, 96.8671)
  line L16 (22.3284, 94.9671) -> (22.3284, 89.42)
  line L17 (8.892, 89.42) -> (8.892, 94.9671)
  arc A44 (65.8, 0) -> (0, 65.8) centre (0, 0) ccw
  arc A45 (172, 65.8) -> (106.2, 0) centre (172, 0) ccw
  arc A46 (106.2, 172) -> (172, 106.2) centre (172, 172) ccw
  arc A47 (0, 106.2) -> (65.8, 172) centre (0, 172) ccw
  line L18 (65.8, 172) -> (68.8, 172)
  line L19 (68.8, 172) -> (68.8, 165.5)
  line L20 (68.8, 165.5) -> (71, 165.5)
  line L21 (71, 165.5) -> (71, 172)
  line L22 (71, 172) -> (72.516, 172)
  line L23 (89.42, 169.948) -> (94.4881, 169.948)
  line L24 (106.2, 172) -> (103.2, 172)
  line L25 (103.2, 172) -> (103.2, 165.5)
  line L26 (103.2, 165.5) -> (101, 165.5)
  line L27 (101, 165.5) -> (101, 172)
  line L28 (101, 172) -> (99.484, 172)
  arc A48 (99.484, 172) -> (99.0181, 171.945) centre (99.484, 170) ccw
  arc A49 (94.4881, 169.948) -> (95.3941, 170.165) centre (94.4881, 171.948) ccw
  arc A50 (99.0181, 171.945) -> (98.5779, 171.783) centre (99.484, 170) ccw
  line L29 (98.5779, 171.783) -> (95.3941, 170.165)
  arc A51 (89.42, 169.948) -> (83.1656, 170.4413) centre (86, 166.482) ccw
  arc A52 (80.8364, 170.4419) -> (83.1656, 170.4413) centre (82.0014, 172.0675) ccw
  arc A53 (80.8364, 170.4419) -> (76.2982, 171.0462) centre (78, 166.484) ccw
  arc A54 (74.6931, 171.1371) -> (76.2982, 171.0462) centre (75.5992, 172.92) ccw
  arc A55 (73.4221, 171.783) -> (72.516, 172) centre (72.516, 170) ccw
  line L30 (73.4221, 171.783) -> (74.6931, 171.1371)
  line L31 (172, 106.2) -> (172, 103.2)
  line L32 (172, 103.2) -> (165.5, 103.2)
  line L33 (165.5, 103.2) -> (165.5, 101)
  line L34 (165.5, 101) -> (172, 101)
  line L35 (172, 101) -> (172, 99.484)
  line L36 (169.948, 82.58) -> (169.948, 77.5119)
  line L37 (172, 65.8) -> (172, 68.8)
  line L38 (172, 68.8) -> (165.5, 68.8)
  line L39 (165.5, 68.8) -> (165.5, 71)
  line L40 (165.5, 71) -> (172, 71)
  line L41 (172, 71) -> (172, 72.516)
  arc A56 (172, 72.516) -> (171.783, 73.4221) centre (170, 72.516) ccw
  arc A57 (169.948, 77.5119) -> (170.165, 76.6059) centre (171.948, 77.5119) ccw
  line L42 (171.783, 73.4221) -> (170.165, 76.6059)
  arc A58 (169.948, 82.58) -> (170.4413, 88.8344) centre (166.482, 86) ccw
  arc A59 (170.4419, 91.1636) -> (170.4413, 88.8344) centre (172.0675, 89.9986) ccw
  arc A60 (170.4419, 91.1636) -> (171.0462, 95.7018) centre (166.484, 94) ccw
  arc A61 (171.1371, 97.3069) -> (171.0462, 95.7018) centre (172.92, 96.4008) ccw
  arc A62 (171.783, 98.5779) -> (172, 99.484) centre (170, 99.484) ccw
  line L43 (171.783, 98.5779) -> (171.1371, 97.3069)
  line L44 (106.2, 0) -> (103.2, 0)
  line L45 (103.2, 0) -> (103.2, 6.5)
  line L46 (103.2, 6.5) -> (101, 6.5)
  line L47 (101, 6.5) -> (101, 0)
  line L48 (101, 0) -> (99.484, 0)
  line L49 (65.8, 0) -> (68.8, 0)
  line L50 (68.8, 0) -> (68.8, 6.5)
  line L51 (68.8, 6.5) -> (71, 6.5)
  line L52 (71, 6.5) -> (71, 0)
  line L53 (71, 0) -> (72.516, 0)
  line L54 (82.58, 2.052) -> (77.5119, 2.052)
  arc A63 (72.516, 0) -> (73.4221, 0.217) centre (72.516, 2) ccw
  arc A64 (77.5119, 2.052) -> (76.6059, 1.835) centre (77.5119, 0.052) ccw
  line L55 (76.6059, 1.835) -> (73.4221, 0.217)
  arc A65 (82.58, 2.052) -> (88.8344, 1.5587) centre (86, 5.518) ccw
  arc A66 (91.1636, 1.5581) -> (88.8344, 1.5587) centre (89.9986, -0.0675) ccw
  arc A67 (91.1636, 1.5581) -> (95.7018, 0.9538) centre (94, 5.516) ccw
  arc A68 (97.3069, 0.8629) -> (95.7018, 0.9538) centre (96.4008, -0.92) ccw
  arc A69 (98.5779, 0.217) -> (99.484, 0) centre (99.484, 2) ccw
  line L56 (98.5779, 0.217) -> (97.3069, 0.8629)
  arc A70 (56.1767, 84.1823) -> (55.8078, 82.0705) centre (57.6556, 82.8359) ccw
  arc A71 (56.1767, 84.1823) -> (56.1767, 87.8177) centre (54.1802, 86) ccw
  arc A72 (55.8078, 89.9295) -> (56.1767, 87.8177) centre (57.6556, 89.1641) ccw
  arc A73 (104.5705, 61.8724) -> (105.803, 63.6265) centre (103.8052, 63.7201) ccw
  arc A74 (108.3735, 66.197) -> (105.803, 63.6265) centre (108.5, 63.5) ccw
  arc A75 (108.3735, 66.197) -> (110.1276, 67.4295) centre (108.2799, 68.1948) ccw
  arc A76 (116.1922, 82.0705) -> (115.8233, 84.1823) centre (114.3444, 82.8359) ccw
  arc A77 (115.8233, 87.8177) -> (115.8233, 84.1823) centre (117.8198, 86) ccw
  arc A78 (115.8233, 87.8177) -> (116.1922, 89.9295) centre (114.3444, 89.1641) ccw
  line L57 (116.1922, 82.0705) -> (110.1276, 67.4295)
  arc A79 (110.1276, 104.5705) -> (108.3735, 105.803) centre (108.2799, 103.8052) ccw
  arc A80 (105.803, 108.3735) -> (108.3735, 105.803) centre (108.5, 108.5) ccw
  arc A81 (105.803, 108.3735) -> (104.5705, 110.1276) centre (103.8052, 108.2799) ccw
  line L58 (110.1276, 104.5705) -> (116.1922, 89.9295)
  arc A82 (89.9295, 116.1922) -> (87.8177, 115.8233) centre (89.1641, 114.3444) ccw
  arc A83 (84.1823, 115.8233) -> (87.8177, 115.8233) centre (86, 117.8198) ccw
  arc A84 (84.1823, 115.8233) -> (82.0705, 116.1922) centre (82.8359, 114.3444) ccw
  line L59 (89.9295, 116.1922) -> (104.5705, 110.1276)
  arc A85 (29.1684, 77.0329) -> (31.0684, 75.1329) centre (31.0684, 77.0329) ccw
  arc A86 (32.9349, 75.1329) -> (33.8405, 75.3626) centre (32.9349, 77.0329) ccw
  arc A87 (41.094, 79.2953) -> (42.0884, 80.9656) centre (40.1884, 80.9656) ccw
  arc A88 (33.8405, 96.6374) -> (32.9349, 96.8671) centre (32.9349, 94.9671) ccw
  arc A89 (42.0884, 91.0344) -> (41.094, 92.7047) centre (40.1884, 91.0344) ccw
  arc A90 (42.0884, 89.42) -> (42.0884, 82.58) centre (45.5084, 86) ccw
  line L60 (29.1684, 82.58) -> (29.1684, 77.0329)
  line L61 (31.0684, 75.1329) -> (32.9349, 75.1329)
  line L62 (33.8405, 75.3626) -> (41.094, 79.2953)
  line L63 (42.0884, 80.9656) -> (42.0884, 82.58)
  line L64 (42.0884, 89.42) -> (42.0884, 91.0344)
  line L65 (41.094, 92.7047) -> (33.8405, 96.6374)
  arc A91 (21.3275, 68.8) -> (23.0414, 65.9031) centre (23.9793, 68.4135) ccw
  arc A92 (28.9832, 63.7004) -> (29.964, 63.5) centre (29.964, 66) ccw
  arc A93 (37.1791, 72.401) -> (35.45, 72.3159) centre (36.4033, 70.5576) ccw
  arc A94 (49.2953, 63.5) -> (49.8761, 65.314) centre (49.2953, 64.5) ccw
  arc A95 (32.2621, 71) -> (33.692, 71.3627) centre (32.2621, 74) ccw
  line L66 (21.3275, 68.8) -> (25.5, 68.8)
  line L67 (25.5, 68.8) -> (25.5, 71)
  line L68 (25.5, 71) -> (32.2621, 71)
  line L69 (33.692, 71.3627) -> (35.45, 72.3159)
  arc A96 (49.8761, 65.314) -> (37.1791, 72.401) centre (11.6541, 11.7536) ccw
  line L70 (49.2953, 63.5) -> (29.964, 63.5)
  arc A97 (28.9832, 63.7004) -> (23.0414, 65.9031) centre (3.1615, 3.1616) ccw
  arc A98 (40.6676, 75.1447) -> (40.7299, 73.3555) centre (41.1442, 74.2656) ccw
  arc A99 (53.2882, 78.848) -> (49.7869, 80.089) centre (50.9785, 77.8913) ccw
  arc A100 (58.1489, 63.5) -> (59.0728, 64.8827) centre (58.1489, 64.5) ccw
  arc A101 (55.928, 63.7361) -> (56.5733, 63.5) centre (56.5733, 64.5) ccw
  arc A102 (55.928, 63.7361) -> (40.7299, 73.3555) centre (13.4685, 13.4685) ccw
  line L71 (56.5733, 63.5) -> (58.1489, 63.5)
  line L72 (59.0728, 64.8827) -> (53.2882, 78.848)
  line L73 (49.7869, 80.089) -> (40.6676, 75.1447)
  arc A103 (49.7869, 91.911) -> (53.2882, 93.152) centre (50.9785, 94.1087) ccw
  arc A104 (40.7299, 98.6445) -> (40.6676, 96.8553) centre (41.1442, 97.7344) ccw
  arc A105 (56.5733, 108.5) -> (55.928, 108.2639) centre (56.5733, 107.5) ccw
  arc A106 (59.0728, 107.1173) -> (58.1489, 108.5) centre (58.1489, 107.5) ccw
  line L74 (56.5733, 108.5) -> (58.1489, 108.5)
  line L75 (59.0728, 107.1173) -> (53.2882, 93.152)
  line L76 (49.7869, 91.911) -> (40.6676, 96.8553)
  arc A107 (40.7299, 98.6445) -> (55.928, 108.2639) centre (13.4685, 158.5315) ccw
  arc A108 (53.3233, 60.5) -> (52.9958, 59.6222) centre (53.3233, 60) ccw
  arc A109 (60.5, 58) -> (58, 60.5) centre (58, 58) ccw
  arc A110 (59.6222, 52.9958) -> (60.5, 53.3233) centre (60, 53.3233) ccw
  line L77 (60.5, 53.3233) -> (60.5, 58)
  arc A111 (59.6222, 52.9958) -> (52.9958, 59.6222) centre (9.8995, 9.8995) ccw
  line L78 (53.3233, 60.5) -> (58, 60.5)
  arc A112 (23.0414, 106.0969) -> (21.3275, 103.2) centre (23.9793, 103.5865) ccw
  arc A113 (29.964, 108.5) -> (28.9832, 108.2996) centre (29.964, 106) ccw
  arc A114 (35.45, 99.6841) -> (37.1791, 99.599) centre (36.4033, 101.4424) ccw
  arc A115 (49.8761, 106.686) -> (49.2953, 108.5) centre (49.2953, 107.5) ccw
  arc A116 (33.692, 100.6373) -> (32.2621, 101) centre (32.2621, 98) ccw
  arc A117 (37.1791, 99.599) -> (49.8761, 106.686) centre (11.6541, 160.2464) ccw
  line L79 (35.45, 99.6841) -> (33.692, 100.6373)
  line L80 (32.2621, 101) -> (25.5, 101)
  line L81 (25.5, 101) -> (25.5, 103.2)
  line L82 (25.5, 103.2) -> (21.3275, 103.2)
  arc A118 (23.0414, 106.0969) -> (28.9832, 108.2996) centre (3.1615, 168.8384) ccw
  line L83 (29.964, 108.5) -> (49.2953, 108.5)
  arc A119 (77.0329, 142.8316) -> (75.1329, 140.9316) centre (77.0329, 140.9316) ccw
  arc A120 (89.42, 149.6716) -> (82.58, 149.6716) centre (86, 146.2516) ccw
  arc A121 (82.58, 142.8316) -> (89.42, 142.8316) centre (86, 146.2516) ccw
  arc A122 (94.9671, 149.6716) -> (96.8671, 151.5716) centre (94.9671, 151.5716) ccw
  arc A123 (75.1329, 151.5716) -> (77.0329, 149.6716) centre (77.0329, 151.5716) ccw
  arc A124 (96.8671, 140.9316) -> (94.9671, 142.8316) centre (94.9671, 140.9316) ccw
  arc A125 (89.42, 129.9116) -> (82.58, 129.9116) centre (86, 126.4916) ccw
  arc A126 (79.2953, 130.906) -> (80.9656, 129.9116) centre (80.9656, 131.8116) ccw
  arc A127 (91.0344, 129.9116) -> (92.7047, 130.906) centre (91.0344, 131.8116) ccw
  arc A128 (96.6374, 138.1595) -> (96.8671, 139.0651) centre (94.9671, 139.0651) ccw
  line L84 (89.42, 129.9116) -> (91.0344, 129.9116)
  line L85 (82.58, 129.9116) -> (80.9656, 129.9116)
  line L86 (77.0329, 142.8316) -> (82.58, 142.8316)
  line L87 (89.42, 142.8316) -> (94.9671, 142.8316)
  line L88 (96.8671, 140.9316) -> (96.8671, 139.0651)
  line L89 (96.6374, 138.1595) -> (92.7047, 130.906)
  line L90 (89.42, 149.6716) -> (94.9671, 149.6716)
  line L91 (82.58, 149.6716) -> (77.0329, 149.6716)
  arc A129 (83.1636, 162.6162) -> (80.8344, 162.6167) centre (81.9986, 160.9905) ccw
  arc A130 (83.1636, 162.6162) -> (89.42, 163.108) centre (86, 166.574) ccw
  arc A131 (96.8671, 161.208) -> (94.9671, 163.108) centre (94.9671, 161.208) ccw
  line L92 (94.9671, 163.108) -> (89.42, 163.108)
  line L93 (96.8671, 161.208) -> (96.8671, 151.5716)
  arc A132 (58, 111.5) -> (60.5, 114) centre (58, 114) ccw
  arc A133 (52.9958, 112.3778) -> (53.3233, 111.5) centre (53.3233, 112) ccw
  arc A134 (60.5, 118.6767) -> (59.6222, 119.0042) centre (60, 118.6767) ccw
  arc A135 (52.9958, 112.3778) -> (59.6222, 119.0042) centre (9.8995, 162.1005) ccw
  line L94 (60.5, 118.6767) -> (60.5, 114)
  line L95 (58, 111.5) -> (53.3233, 111.5)
  arc A136 (63.7361, 116.072) -> (63.5, 115.4267) centre (64.5, 115.4267) ccw
  arc A137 (63.5, 113.8511) -> (64.8827, 112.9272) centre (64.5, 113.8511) ccw
  arc A138 (78.848, 118.7118) -> (80.089, 122.2131) centre (77.8913, 121.0215) ccw
  arc A139 (75.1447, 131.3324) -> (73.3555, 131.2701) centre (74.2656, 130.8558) ccw
  line L96 (80.089, 122.2131) -> (75.1447, 131.3324)
  line L97 (78.848, 118.7118) -> (64.8827, 112.9272)
  line L98 (63.5, 113.8511) -> (63.5, 115.4267)
  arc A140 (63.7361, 116.072) -> (73.3555, 131.2701) centre (13.4685, 158.5315) ccw
  arc A141 (63.5, 122.7047) -> (65.314, 122.1239) centre (64.5, 122.7047) ccw
  arc A142 (71, 139.7379) -> (71.3627, 138.308) centre (74, 139.7379) ccw
  arc A143 (72.401, 134.8209) -> (72.3159, 136.55) centre (70.5576, 135.5967) ccw
  arc A144 (63.7004, 143.0168) -> (63.5, 142.036) centre (66, 142.036) ccw
  arc A145 (68.8, 150.6725) -> (65.9031, 148.9586) centre (68.4135, 148.0207) ccw
  arc A146 (65.314, 122.1239) -> (72.401, 134.8209) centre (11.7536, 160.3459) ccw
  line L99 (72.3159, 136.55) -> (71.3627, 138.308)
  line L100 (63.5, 122.7047) -> (63.5, 142.036)
  line L101 (68.8, 146.5) -> (71, 146.5)
  line L102 (71, 146.5) -> (71, 139.7379)
  line L103 (68.8, 146.5) -> (68.8, 150.6725)
  arc A147 (63.7004, 143.0168) -> (65.9031, 148.9586) centre (3.1615, 168.8384) ccw
  arc A148 (38.545, 113.3432) -> (39.0827, 111.5) centre (39.0827, 112.5) ccw
  arc A149 (48.0955, 111.5) -> (49.3372, 111.9321) centre (48.0955, 113.5) ccw
  arc A150 (60.0679, 122.6628) -> (60.5, 123.9045) centre (58.5, 123.9045) ccw
  arc A151 (60.5, 132.9173) -> (58.6568, 133.455) centre (59.5, 132.9173) ccw
  line L104 (60.5, 132.9173) -> (60.5, 123.9045)
  line L105 (39.0827, 111.5) -> (48.0955, 111.5)
  arc A152 (38.545, 113.3432) -> (58.6568, 133.455) centre (3.1615, 168.8384) ccw
  arc A153 (49.3372, 111.9321) -> (60.0679, 122.6628) centre (8.4853, 163.5147) ccw
  arc A154 (108.5, 115.4267) -> (108.2639, 116.072) centre (107.5, 115.4267) ccw
  arc A155 (107.1173, 112.9272) -> (108.5, 113.8511) centre (107.5, 113.8511) ccw
  arc A156 (98.6445, 131.2701) -> (96.8553, 131.3324) centre (97.7344, 130.8558) ccw
  arc A157 (98.6445, 131.2701) -> (108.2639, 116.072) centre (158.5315, 158.5315) ccw
  line L106 (108.5, 115.4267) -> (108.5, 113.8511)
  line L107 (91.911, 122.2131) -> (96.8553, 131.3324)
  arc A158 (106.0968, 148.9586) -> (103.2, 150.6725) centre (103.5865, 148.0207) ccw
  arc A159 (108.5, 142.036) -> (108.2996, 143.0168) centre (106, 142.036) ccw
  arc A160 (99.6841, 136.55) -> (99.599, 134.8209) centre (101.4423, 135.5967) ccw
  arc A161 (100.6373, 138.308) -> (101, 139.7379) centre (98, 139.7379) ccw
  arc A162 (106.686, 122.1239) -> (108.5, 122.7047) centre (107.5, 122.7047) ccw
  arc A163 (106.0968, 148.9586) -> (108.2996, 143.0168) centre (168.8384, 168.8384) ccw
  arc A164 (99.599, 134.8209) -> (106.686, 122.1239) centre (160.2464, 160.3459) ccw
  line L108 (99.6841, 136.55) -> (100.6373, 138.308)
  line L109 (101, 139.7379) -> (101, 146.5)
  line L110 (101, 146.5) -> (103.2, 146.5)
  line L111 (103.2, 146.5) -> (103.2, 150.6725)
  line L112 (108.5, 142.036) -> (108.5, 122.7047)
  arc A165 (111.5, 114) -> (114, 111.5) centre (114, 114) ccw
  arc A166 (118.6767, 111.5) -> (119.0041, 112.3778) centre (118.6767, 112) ccw
  arc A167 (112.3778, 119.0042) -> (111.5, 118.6767) centre (112, 118.6767) ccw
  arc A168 (112.3778, 119.0042) -> (119.0041, 112.3778) centre (162.1005, 162.1005) ccw
  line L113 (114, 111.5) -> (118.6767, 111.5)
  line L114 (111.5, 114) -> (111.5, 118.6767)
  arc A169 (111.5, 123.9045) -> (111.9321, 122.6628) centre (113.5, 123.9045) ccw
  arc A170 (113.3431, 133.4551) -> (111.5, 132.9173) centre (112.5, 132.9173) ccw
  arc A171 (132.9173, 111.5) -> (133.455, 113.3432) centre (132.9173, 112.5) ccw
  arc A172 (122.6628, 111.9321) -> (123.9045, 111.5) centre (123.9045, 113.5) ccw
  arc A173 (111.9321, 122.6628) -> (122.6628, 111.9321) centre (163.5147, 163.5147) ccw
  arc A174 (113.3431, 133.4551) -> (133.5298, 113.2905) centre (168.9085, 168.8947) ccw
  line L115 (123.9045, 111.5) -> (132.9173, 111.5)
  line L116 (111.5, 123.9045) -> (111.5, 132.9173)
  arc A175 (116.072, 108.2639) -> (115.4267, 108.5) centre (115.4267, 107.5) ccw
  arc A176 (113.8511, 108.5) -> (112.9272, 107.1173) centre (113.8511, 107.5) ccw
  arc A177 (131.3324, 96.8553) -> (131.2701, 98.6445) centre (130.8558, 97.7344) ccw
  arc A178 (118.7118, 93.152) -> (122.2131, 91.911) centre (121.0215, 94.1087) ccw
  arc A179 (116.072, 108.2639) -> (131.2701, 98.6445) centre (158.5315, 158.5315) ccw
  line L117 (122.2131, 91.911) -> (131.3324, 96.8553)
  line L118 (113.8511, 108.5) -> (115.4267, 108.5)
  line L119 (112.9272, 107.1173) -> (118.7118, 93.152)
  arc A180 (150.6725, 103.2) -> (148.9586, 106.0969) centre (148.0207, 103.5865) ccw
  arc A181 (143.0168, 108.2996) -> (142.036, 108.5) centre (142.036, 106) ccw
  arc A182 (134.8209, 99.599) -> (136.55, 99.6841) centre (135.5967, 101.4424) ccw
  arc A183 (139.7379, 101) -> (138.308, 100.6373) centre (139.7379, 98) ccw
  arc A184 (122.7047, 108.5) -> (122.1239, 106.686) centre (122.7047, 107.5) ccw
  line L120 (122.7047, 108.5) -> (142.036, 108.5)
  line L121 (146.5, 103.2) -> (150.6725, 103.2)
  line L122 (146.5, 103.2) -> (146.5, 101)
  line L123 (146.5, 101) -> (139.7379, 101)
  line L124 (138.308, 100.6373) -> (136.55, 99.6841)
  arc A185 (122.1239, 106.686) -> (134.8209, 99.599) centre (160.3459, 160.2464) ccw